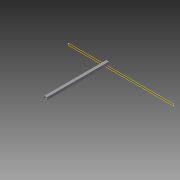
# Autodesk Inventor part: StaticForks
Saved by Autodesk Inventor 2015 (Build 190159000, 159)
## iProperties
Created: 2015-01-25
Part Number: StaticForks
Material: Generic
Document SubType Name: Modeling
Designer: jhirshland1
Density: 1 g/cm^3
Appearance: Default
Author: jhirshland1
Autodesk Inventor part; units mm, degrees
ref_plane "YZ Plane" through (0, 0, 0) normal (1, 0, 0) x (0, 1, 0)
ref_plane "XZ Plane" through (0, 0, 0) normal (0, 1, 0) x (-1, 0, 0)
ref_plane "XY Plane" through (0, 0, 0) normal (0, 0, 1) x (1, 0, 0)
ref_plane "Work Plane1" through (-350.1142, 119.2278, 28.1686) normal (0, 0, 1) x (0, 1, 0)
sketch "Sketch1" plane through (-350.1142, 119.2278, 28.1686) normal (0, 0, 1) x (0, 1, 0)
  line L0 (70.9812, -246.6013) -> (51.9312, -246.6013)
  line L1 (51.9312, -246.6013) -> (51.9312, -265.6513)
  line L2 (51.9312, -265.6513) -> (70.9812, -265.6513)
  line L3 (70.9812, -265.6513) -> (70.9812, -246.6013)
  line L4 (67.8062, -249.7763) -> (55.1062, -249.7763)
  line L5 (55.1062, -249.7763) -> (55.1062, -262.4763)
  line L6 (55.1062, -262.4763) -> (67.8062, -262.4763)
  line L7 (67.8062, -262.4763) -> (67.8062, -249.7763)
  point P0 (-119.2278, -350.1142)
  dimension "d0" = 19.05
  dimension "d1" = 19.05
  dimension "d2" = 3.175
  constraints: 16 end point, 4 parallel, 2 perpendicular, 1 horizontal, 3 other
  measures "d0" distance of L2.end L1.end
  measures "d1" distance of L1.end L0.end
  measures "d2" distance between parallel lines of L3 L7
extrude "Extrusion1" add sketch "Sketch1" along normal blind 457.2
body "Solid1"
